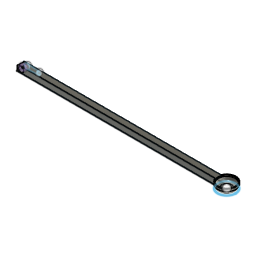
Catapult Arm v2 (Autodesk Fusion 360 design; units mm, degrees)
Autodesk Fusion 360 part; units mm, degrees
sketch "Sketch1" plane through (0, 0, 0) normal (0, 0, 1) x (1, 0, 0)
  line L0 (0, 0) -> (280, 0)
  line L1 (280, 0) -> (280, -8)
  line L2 (280, -8) -> (0, -8)
  line L3 (0, -8) -> (0, 0)
  dimension "d1" = 280
  dimension "d2" = 8
  constraint horizontal L0
  constraint vertical L1
  constraint horizontal L2
  constraint vertical L3
  constraint coincident L0.start L3.end
  measures "d1" distance of L0.start L0.end
  measures "d2" distance of L0.start L2.end
extrude "Extrude1" add sketch "Sketch1" along normal blind 8
sketch "Sketch2" plane through (0, 0, 0) normal (0, 0, 1) x (1, 0, 0)
  circle A0 centre (280, -4) radius 12.5
  circle A1 centre (280, -4) radius 11.3
  dimension "d5" = 25
  dimension "d6" = 22.6
  constraint concentric A0 A1
  measures "d5" diameter of A0
  measures "d6" diameter of A1
extrude "Extrude2" add sketch "Sketch2" along normal blind 8
extrude "Extrude3" cut sketch "Sketch2" along normal blind 8 contours A1
extrude "Extrude4" add sketch "Sketch2" along normal blind 1.2 contours A1
fillet "Fillet1" radius 5 1 edges at (269.4647, 0.0863, 1.2)
sketch "Sketch4" plane through (0, 0, 0) normal (0, 1, 0) x (-1, 0, 0)
  line L0 (-268.1573, 8) -> (-268.1573, 0)
  line L1 (-268.1573, 0) -> (0, 0)
  line L2 (0, 0) -> (0, 8)
  line L3 (0, 8) -> (-268.1573, 8)
  circle A0 centre (-5.4, 4.0245) radius 3.45
  circle A1 centre (-21.4, 3.9983) radius 2.05
  line L4 (-21.5827, 6.0402) -> (-5.7075, 7.4608)
  line L5 (-5.6963, 0.5873) -> (-21.576, 1.9559)
  dimension "d20" = 6.9
  dimension "d21" = 5.4
  dimension "d22" = 4.1
  dimension "d23" = 16
  constraint coincident A1 L4.start
  constraint coincident A0 L4.end
  constraint coincident A0 L5.start
  constraint coincident A1 L5.end
  constraint tangent A1 L5
  constraint tangent A1 L4
  constraint tangent A0 L4
  constraint tangent A0 L5
  measures "d20" diameter of A0
  measures "d21" distance of L2 A0.centre
  measures "d22" diameter of A1
  measures "d23" horizontal distance of A0.centre A1.centre
extrude "Extrude5" cut sketch "Sketch4" against normal blind 6 contours A0 | A0 A1 L4 L5 | A1
extrude "Extrude6" cut sketch "Sketch4" against normal blind 8 contours A0
fillet "Fillet2" radius 5 1 edges at (292.5, -4, 0)
fillet "Fillet3" radius 2 1 edges at (0, -4, 8)
fillet "Fillet4" radius 2 1 edges at (0, -4, 0)
equation "d6 = 25 mm - ( 1.2 * 2 ) * 1 mm"
equation "d21 = 3.4 mm + 2 mm"
